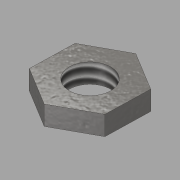
# Autodesk Inventor part: Electronics Mounting nut
Saved by Autodesk Inventor 2017 (Build 210142000, 142)
## iProperties
Created: 2017-01-17
Part Number: Electronics Mounting nut
Material: Steel, Galvanized
Document SubType Name: Modeling
Designer: qupec
Density: 7.85 g/cm^3
Appearance: Galvanized
Author: qupec
Autodesk Inventor part; units mm, degrees
ref_plane "YZ Plane" through (0, 0, 0) normal (1, 0, 0) x (0, 1, 0)
ref_plane "XZ Plane" through (0, 0, 0) normal (0, 1, 0) x (-1, 0, 0)
ref_plane "XY Plane" through (0, 0, 0) normal (0, 0, 1) x (1, 0, 0)
sketch "Sketch1" plane through (0, 0, 0) normal (0, 1, 0) x (-1, 0, 0)
  line L0 (2.5744, 1.4052) -> (2.5041, -1.5269)
  line L1 (2.5041, -1.5269) -> (-0.0703, -2.9321)
  line L2 (-0.0703, -2.9321) -> (-2.5744, -1.4052)
  line L3 (-2.5744, -1.4052) -> (-2.5041, 1.5269)
  line L4 (-2.5041, 1.5269) -> (0.0703, 2.9321)
  line L5 (0.0703, 2.9321) -> (2.5744, 1.4052)
  circle A0 centre (0, 0) radius 1.3589
  dimension "d0" = 2.7178
  dimension "d1" = 5.08
  constraints: 12 end point, 2 coincident, 1 centre point, 13 other
  measures "d0" diameter of A0
  measures "d1" distance between parallel lines of L3 L0
extrude "Extrusion1" add sketch "Sketch1" along normal blind 1.27
thread "Thread1" size "4-40 UNC" class "2B" standard "ANSI Unified Screw Threads" full length
body "Solid1"
